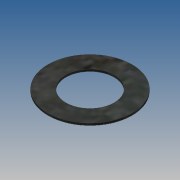
# Autodesk Inventor part: Unterlegescheibe_ra8846s
Saved by Autodesk Inventor 2021 (Build 250183000, 183)
## iProperties
Created: 2020-11-16
Part Number: Unterlegescheibe_ra8846s
Material: Stahl
Document SubType Name: Modeling
Designer: Ricardo A
Density: 7.85 g/cm^3
Appearance: Platte
Description: motor_teil2_scheibe
Mass: 0.4226 g
Surface Area: 3.00839 cm^2
Volume: 0.0538343 cm^3
Author: Ricardo A
Title: Unterlegscheibe
Revision Number: Rev00
Autodesk Inventor part; units mm, degrees
ref_plane "YZ-Ebene" through (0, 0, 0) normal (1, 0, 0) x (0, 1, 0)
ref_plane "XZ-Ebene" through (0, 0, 0) normal (0, 1, 0) x (-1, 0, 0)
ref_plane "XY-Ebene" through (0, 0, 0) normal (0, 0, 1) x (1, 0, 0)
sketch "Skizze1" plane through (0, 0, 0) normal (0, 0, 1) x (1, 0, 0)
  line L0 (-11.2, 0) -> (11.2, 0) projected
  line L1 (0, -11.2) -> (0, 11.2) projected
  circle A0 centre (0, 0) radius 4.6
  circle A1 centre (0, 0) radius 8
  dimension "d0" = 9.2
  dimension "d1" = 16
  constraints: 2 centre point, 2 coincident
  measures "d0" diameter of A0
  measures "d1" diameter of A1
extrude "Extrusion1" add sketch "Skizze1" along normal blind 0.4 contours A0 L1 A1 L0 | L0 A1 L1 A0 | A0 L0 A1 L1 | L1 A1 L0 A0
